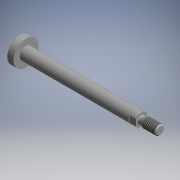
# Autodesk Inventor part: 536218 ADN-50-P-A_(KS)
Saved by Autodesk Inventor 2017.3 (Build 213256000, 256)
## iProperties
Part Number: 536218 ADN-50-P-A_(KS)
Material: Generic
Catalog Web Link: www.cadenas.de
Description: ADN-(KS)-Compact cylinder - piston rod
Vendor: FESTO
Document SubType Name: Modeling
Designer: partserver
Manufacturer: FESTO
Mass: 4.80589 g
Surface Area: 26.7319 cm^2
Volume: 4.80589 cm^3
Density: 1 g/cm^3
Appearance: PSOLRGB-191-191-191
Category: PARTsolutions
Company: FESTO
Title: 536218 ADN-50-P-A_(KS)
Author: Cadenas PARTsolutions
Comments: Compact cylinder - piston rod
PSOL_IDENT_0: {$CADENAS_DATA\23d-libs\festo\parts\a\adn\parts\adn_ks.prj},236 {VTYP=3D},{NB=536218 ADN-50-P-A_(KS)
PSOL_IDENT_1: },{LINA=536218 ADN-50-P-A_(KS)},{NN=ADN-(KS)},{DATE=20.11.2019 12:35:12},{GEOMDATE=08.01.2019 14:34:
PSOL_IDENT_2: 57},{VERSION=},{LINEID=8180},{WBVAR=DF,HUB,TH,Q,S2S20,K2,K5,K8,K10,S1,TT,R8},{WBNUMERIC=HUB,K2,K8}
PSOL_IDENT_3: {NB=536218 ADN-50-P-A_(KS)},{LINA=536218 ADN-50-P-A_(KS)},{KT=536218},{TNR=536218},{AUSF=ADN},{DF=P}
PSOL_IDENT_4: ,{GA=A},{WHX=4.7},{WH0=4.700},{WH1=0.000},{WH2=0.000},{WH3=0.000},{WHX1=4.7},{WHX2=5.35},{WH=4.7},{Z
PSOL_IDENT_5: M=45.700},{ZM2=0.000},{ZB=39.700},{ZB1=0.000},{ZB2=0.000},{ZB6=0.000},{ZA=35.000},{KDM=16},{HUBP=-},
PSOL_IDENT_6: {HUB=50},{HUB1=[1-300]},{HUB2=[1-200]},{HUB3=0},{HUB4=0},{TH=A},{THC='A','I'},{Q=-},{VAR1C='-','Q'},
PSOL_IDENT_7: {S2S20=-},{VAR2C='-','S2','S20'},{VAR22C='-','S2'},{VAR222C='-','S2','S20'},{K2=0},{VAR3C=0,[1-10]},
PSOL_IDENT_8: {VAR33C=0,[1-10]},{K5=-},{K5A='-','M8'},{K5I='-'},{K5S1A='-'},{K5S1I='-'},{K5C='-','M8'},{K5N=0},{K5
PSOL_IDENT_9: P=0},{K5T=},{K8=0},{K10=-},{K10A='-'},{K10N=},{S1=-},{TT=-},{TT1='-'},{R8=-},{R81='-'},{VAR4C=0,[1-3
PSOL_IDENT_10: 00]},{VAR5C='-','S6'},{VAR6C='-'},{VAR66C='-'},{VAR7C='-','R3'},{HUBALG=[1-300]},{A=12.000},{A1=0.00
PSOL_IDENT_11: 0},{AF=10.000},{AF1=0.000},{AF2=10.000},{AF3=0.000},{AF5=0.000},{AF7=0.000},{D8=3.200},{D9=4.500},{K
PSOL_IDENT_12: F=M4},{KFN=4.000},{KF1=-},{KF1C=0.0000},{KF2=-},{KF2C=0.0000},{KF3=M4},{KF3C=4.0000},{KF5=-},{KF5N=0
PSOL_IDENT_13: },{KF7=-},{KF7N=0},{KK=M6},{KKN=6},{KKP=1.00},{KK1=-},{KK1N=0.0000},{KK1P=0.00},{L2=35.000},{L8=3.00
PSOL_IDENT_14: 0},{MM=8.000},{MM1=0.000},{PL=6.000},{SF=7},{SF1=0},{SF3=7.0},{WL=3.700},{WL1=0.000},{QN=},{S2N=},{S
PSOL_IDENT_15: 1N=},{K2N=},{K8N=},{KKC3=4.500},{KKF2=0.400},{KKD5=1.300},{KKE2=20.000},{K5C3=0},{K5F2=0},{K5D5=0},{
PSOL_IDENT_16: KK1C3=0.000},{KK1F2=0.000},{KK1D5=0.000},{KK1E2=0.000},{L100S1=0.000},{L101S1=0.000},{L102S1=0.000},
PSOL_IDENT_17: {L103S1=0.000},{D100S1=0.000},{L100=0.400},{L101=1.500},{L102=10.000},{L103=13.000},{D100=4.300},{L1
PSOL_IDENT_18: 00Q=0.400},{L101Q=1.500},{L101K5=1.500},{L102Q=10.000},{L103Q=13.000},{D100Q=4.300},{L100S1K5=0.000}
PSOL_IDENT_19: ,{L101S1K5=0.000},{L102S1K5=0.000},{L103S1K5=0.000},{D100S1K5=0.000},{VERS=1},{TTN=},{R8N=},{D20=0.0
PSOL_IDENT_20: 00},{XF31=3.000},{B31=3.200},{DFALG='P'}
NB: 536218 ADN-50-P-A_(KS)
NN: ADN-(KS)
NT: Compact cylinder - piston rod
NBSYN: $TNR. $AUSF.-$HUB.-$DF.-$TH.$QN.$S2N.$K2N.$K5T.$K8N.$K10N.$S1N.$TTN.$R8N._(KS)
LINA: 536218 ADN-50-P-A_(KS)
CATALOG: Festo
TNR: 536218
AUSF: ADN
DF: P
GA: A
WHX: 4.7
WH0: 4.7
WH1: 0
WH2: 0
WH3: 0
WHX1: 4.7
WHX2: 5.35
WH: 4.7
ZM: 45.7
ZM2: 0
ZB: 39.7
ZB1: 0
ZB2: 0
ZB6: 0
ZA: 35
KDM: 16
HUBP: -
HUB: 50
TH: A
Q: -
S2S20: -
K2: 0
K5: -
K8: 0
K10: -
S1: -
TT: -
R8: -
A: 12
A1: 0
AF: 10
AF1: 0
AF2: 10
AF3: 0
AF5: 0
AF7: 0
D8: 3.2
D9: 4.5
KF: M4
KF1: -
KF2: -
KF3: M4
KF5: -
KF7: -
KK: M6
KK1: -
L2: 35
L8: 3
MM: 8
MM1: 0
PL: 6
SF: 7
SF1: 0
SF3: 7
WL: 3.7
WL1: 0
L101K5: 1.5
D20: 0
XF31: 3
B31: 3.2
SUPPLIER: FESTO
ARTICLENO: 536218 ADN-50-P-A_(KS)
BOMINFO: 536218 ADN-50-P-A_(KS)
CREATOR: CADENAS GmbH
Autodesk Inventor part; units mm, degrees
sketch "Sketch_1" plane through (0, 0, 0) normal (0, 0, 1) x (1, 0, 0)
  line L0 (73, 0) -> (-4.7, 0)
  line L1 (-4.7, 0) -> (-4.7, 4)
  line L2 (-4.7, 4) -> (73, 4)
  line L3 (73, 4) -> (73, 0)
  line L4 (73, 0) -> (-4.7, 0)
  constraints: 10 end point
revolve "Revolution1" add sketch "Sketch_1" angle 360 about axis through (73, 0, 0) along (1, 0, 0)
sketch "Sketch_11" plane through (0, 0, 0) normal (0, 0, 1) x (1, 0, 0)
  line L0 (73, 0) -> (69, 0)
  line L1 (69, 0) -> (69, 8)
  line L2 (69, 8) -> (73, 8)
  line L3 (73, 8) -> (73, 0)
  line L4 (73, 0) -> (69, 0)
  constraints: 10 end point
revolve "Revolution2" add sketch "Sketch_11" angle 360 about axis through (73, 0, 0) along (1, 0, 0)
sketch "Sketch_19" plane through (0, 0, 0) normal (0, 0, 1) x (1, 0, 0)
  line L0 (-3.7, 0) -> (-16.7, 0)
  line L1 (-16.7, 0) -> (-16.7, 2.3865)
  line L2 (-16.7, 2.3865) -> (-16.0865, 3)
  line L3 (-16.0865, 3) -> (-8.0606, 3)
  line L4 (-8.0606, 3) -> (-6.0663, 2.2741)
  arc A0 (-6.0663, 2.2741) -> (-5.9295, 2.25) centre (-5.9295, 2.65) ccw
  line L5 (-5.9295, 2.25) -> (-5.1, 2.25)
  arc A1 (-5.1, 2.25) -> (-4.7, 2.65) centre (-5.1, 2.65) ccw
  line L6 (-4.7, 2.65) -> (-4.7, 3)
  line L7 (-4.7, 3) -> (-3.7, 3)
  line L8 (-3.7, 3) -> (-3.7, 0)
  line L9 (-3.7, 0) -> (-16.7, 0)
  constraints: 20 end point, 4 point on circle, 2 centre point
revolve "Revolution3" add sketch "Sketch_19" angle 360 about axis through (-3.7, 0, 0) along (1, 0, 0)
thread "Thread1" size "M6x1" class "6g" standard "ISO Metric profile" full length
sketch "Sketch_20" plane through (0, 0, 0) normal (0, 0, 1) x (1, 0, 0)
  line L0 (-26.4, -12.5) -> (4.1962, -12.5)
  line L1 (4.1962, -12.5) -> (-1, -3.5)
  line L2 (-1, -3.5) -> (-4.7, -3.5)
  line L3 (-4.7, -3.5) -> (-4.7, -8.5)
  line L4 (-4.7, -8.5) -> (-21.7, -8.5)
  line L5 (-21.7, -8.5) -> (-21.7, 8.5)
  line L6 (-21.7, 8.5) -> (-4.7, 8.5)
  line L7 (-4.7, 8.5) -> (-4.7, 3.5)
  line L8 (-4.7, 3.5) -> (-1, 3.5)
  line L9 (-1, 3.5) -> (4.1962, 12.5)
  line L10 (4.1962, 12.5) -> (-26.4, 12.5)
  line L11 (-26.4, 12.5) -> (-26.4, -12.5)
  constraints: 24 end point
extrude "Extrusion1" cut sketch "Sketch_20" along normal mid plane 16
ref_plane "FDT_PIRODACC_M1_XY" through (-10.9, 0, 0) normal (-1, 0, 0) x (0, 1, 0)
ref_plane "FDT_PIRODACC_M1_YZ" through (-10.9, 0, 0) normal (0, 1, 0) x (0, 0, -1)
ref_plane "FDT_PIRODACC_M1_ZX" through (-10.9, 0, 0) normal (0, 0, -1) x (-1, 0, 0)
ref_plane "NUT1_XY" through (-9.3, 0, 0) normal (1, 0, 0) x (0, 0, -1)
ref_plane "NUT1_YZ" through (-9.3, 0, 0) normal (0, 0, -1) x (0, 1, 0)
ref_plane "NUT1_ZX" through (-9.3, 0, 0) normal (0, 1, 0) x (1, 0, 0)
ref_plane "PISTON_XY" through (73, 0, 0) normal (1, 0, 0) x (0, 0, -1)
ref_plane "PISTON_YZ" through (73, 0, 0) normal (0, 0, -1) x (0, 1, 0)
ref_plane "PISTON_ZX" through (73, 0, 0) normal (0, 1, 0) x (1, 0, 0)
body "Solid1"
